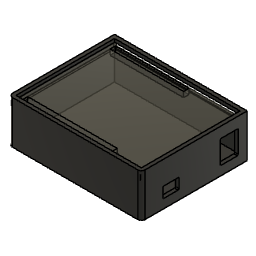
Boite Arduino SATRAGNO (Autodesk Fusion 360 design; units mm, degrees)
Autodesk Fusion 360 part; units mm, degrees
note: some values were not read from the file. Set by a fixed rule: which sketch regions a step uses.
sketch "Esquisse1" plane through (0, 0, 0) normal (0, 1, 0) x (1, 0, 0)
  line L0 (47.3891, -62.8881) -> (-22.6109, -62.8881)
  line L1 (-24.6109, -60.8881) -> (-24.6109, -3.8881)
  line L2 (-24.6109, -3.8881) -> (49.3891, -3.8881)
  line L3 (49.3891, -3.8881) -> (49.3891, -60.8881)
  line L4 (-22.6109, -5.8881) -> (47.3891, -5.8881)
  line L5 (47.3891, -60.8881) -> (-22.6109, -60.8881)
  arc A0 (47.3891, -62.8881) -> (49.3891, -60.8881) centre (47.3891, -60.8881) ccw
  arc A1 (-24.6109, -60.8881) -> (-22.6109, -62.8881) centre (-22.6109, -60.8881) ccw
  line L6 (-22.6109, -5.8881) -> (-22.6109, -60.8881)
  line L7 (47.3891, -5.8881) -> (47.3891, -60.8881)
  point P0 (49.3891, -62.8881)
  point P1 (-24.6109, -62.8881)
  dimension "LongeurCarte" = 74
  dimension "LargeurCrate" = 59
  dimension "d66" = 2
  dimension "d67" = 2
  constraint horizontal L0
  constraint vertical L1
  constraint horizontal L2
  constraint vertical L3
  constraint coincident P0 L0
  constraint coincident P0 L3
  constraint tangent L0 A0
  constraint tangent L3 A0
  constraint coincident P1 L0
  constraint coincident P1 L1
  constraint tangent L0 A1
  constraint tangent L1 A1
  constraint perpendicular L5 L6
  constraint coincident L5.start A0.centre
  constraint perpendicular L5 L7
  measures "LongeurCarte" distance of P0 P1
  measures "LargeurCrate" distance of P1 L1.end
  measures "d66" radius of A0
  measures "d67" radius of A1
extrude "Extrusion5" add sketch "Esquisse1" along normal blind 3 contours L4 L5 L6 L7 makes body 1
extrude "Extrusion6" add sketch "Esquisse1" along normal blind 24 bodies 1
sketch "Esquisse3" plane through (49.3891, 0, 0) normal (1, 0, 0) x (0, 0, -1)
  line L0 (-60.8881, 0) -> (-3.8881, 0)
  line L1 (-3.8881, 0) -> (-3.8881, 24)
  line L2 (-3.8881, 24) -> (-60.8881, 24)
  line L3 (-18.3881, 5) -> (-9.3881, 5)
  line L4 (-18.8881, 5) -> (-18.8881, 0) construction
  line L5 (-18.8881, 5.5) -> (-18.8881, 17.5)
  line L6 (-18.3881, 18) -> (-9.3881, 18)
  line L7 (-8.8881, 17.5) -> (-8.8881, 5.5)
  line L8 (-62.8881, 5) -> (-50.8881, 5) construction
  line L9 (-50.3881, 5) -> (-42.3881, 5)
  line L10 (-3.8881, 0) -> (-60.8881, 0)
  line L11 (-41.8881, 5.5) -> (-41.8881, 10.5)
  line L12 (-42.3881, 11) -> (-50.3881, 11)
  line L13 (-50.8881, 10.5) -> (-50.8881, 5.5)
  arc A0 (-18.3881, 18) -> (-18.8881, 17.5) centre (-18.3881, 17.5) ccw
  arc A1 (-8.8881, 17.5) -> (-9.3881, 18) centre (-9.3881, 17.5) ccw
  arc A2 (-9.3881, 5) -> (-8.8881, 5.5) centre (-9.3881, 5.5) ccw
  arc A3 (-18.8881, 5.5) -> (-18.3881, 5) centre (-18.3881, 5.5) ccw
  arc A4 (-41.8881, 10.5) -> (-42.3881, 11) centre (-42.3881, 10.5) ccw
  arc A5 (-42.3881, 5) -> (-41.8881, 5.5) centre (-42.3881, 5.5) ccw
  arc A6 (-50.8881, 5.5) -> (-50.3881, 5) centre (-50.3881, 5.5) ccw
  arc A7 (-50.3881, 11) -> (-50.8881, 10.5) centre (-50.3881, 10.5) ccw
  line L14 (-60.8881, 24) -> (-60.8881, 0)
  point P0 (-3.8881, 5)
  point P1 (-18.8881, 18)
  point P2 (-8.8881, 18)
  point P3 (-41.8881, 5)
  point P4 (-41.8881, 11)
  point P5 (-50.8881, 11)
  dimension "d18" = 15
  dimension "d19" = 5
  dimension "d20" = 13
  dimension "d21" = 10
  dimension "d22" = 12
  dimension "d23" = 9
  dimension "d24" = 5
  dimension "d25" = 6
  dimension "d26" = 9
  dimension "d27" = 0.5
  dimension "d28" = 0.5
  dimension "d29" = 0.5
  dimension "d30" = 0.5
  dimension "d31" = 0.5
  dimension "d32" = 0.5
  dimension "d33" = 0.5
  dimension "d34" = 0.5
  constraint coincident L1 P0
  constraint perpendicular L1 L3
  constraint coincident L0 L4.end
  constraint perpendicular L0 L4
  constraint perpendicular L3 L5
  constraint perpendicular L5 L6
  constraint perpendicular L3 L7
  constraint perpendicular L9 L11
  constraint perpendicular L11 L12
  constraint coincident P1 L5
  constraint coincident P1 L6
  constraint tangent L5 A0
  constraint tangent L6 A0
  constraint coincident P2 L6
  constraint coincident P2 L7
  constraint tangent L6 A1
  constraint tangent L7 A1
  constraint coincident P0 L3
  constraint tangent L3 A2
  constraint tangent L7 A2
  constraint coincident L4.start L5
  constraint coincident L4.start L3
  constraint tangent L5 A3
  constraint tangent L3 A3
  constraint coincident P4 L12
  constraint coincident P4 L11
  constraint tangent L12 A4
  constraint tangent L11 A4
  constraint coincident P3 L11
  constraint coincident P3 L9
  constraint tangent L11 A5
  constraint tangent L9 A5
  constraint coincident L8.end L13
  constraint coincident L8.end L9
  constraint tangent L13 A6
  constraint tangent L9 A6
  constraint coincident P5 L12
  constraint coincident P5 L13
  constraint tangent L12 A7
  constraint tangent L13 A7
  measures "d18" distance of L4.start P0
  measures "d19" distance of L4.start L4.end
  measures "d20" distance of L4.start P1
  measures "d21" distance of P1 P2
  measures "d22" distance of L8.start L8.end
  measures "d23" distance of L8.end P3
  measures "d24" distance of P3 L10
  measures "d25" distance of P3 P4
  measures "d26" distance of P4 P5
  measures "d27" radius of A0
  measures "d28" radius of A1
  measures "d29" radius of A2
  measures "d30" radius of A3
  measures "d31" radius of A4
  measures "d32" radius of A5
  measures "d33" radius of A6
  measures "d34" radius of A7
extrude "Extrusion7" cut sketch "Esquisse3" against normal blind 2 contours L3 L5 L6 L7 A0 A1 A2 A3 | L9 L11 L12 L13 A4 A5 A6 A7 bodies 1
sketch "Esquisse4" plane through (0, 0, 0) normal (0, 1, 0) x (1, 0, 0)
  line L0 (-73.5353, -62.2391) -> (-145.5353, -62.2391)
  line L1 (-145.5353, -62.2391) -> (-145.5353, -5.2391)
  line L2 (-145.5353, -5.2391) -> (-73.5353, -5.2391)
  line L3 (-73.5353, -5.2391) -> (-73.5353, -62.2391)
  line L4 (-142.5353, -7.2391) -> (-101.5353, -7.2391)
  line L5 (-101.5353, -7.2391) -> (-101.5353, -10.2391)
  line L6 (-101.5353, -10.2391) -> (-142.5353, -10.2391)
  line L7 (-142.5353, -10.2391) -> (-142.5353, -7.2391)
  line L8 (-142.5353, -59.2391) -> (-92.5353, -59.2391)
  line L9 (-92.5353, -59.2391) -> (-92.5353, -56.2391)
  line L10 (-92.5353, -56.2391) -> (-142.5353, -56.2391)
  line L11 (-142.5353, -56.2391) -> (-142.5353, -59.2391)
  dimension "d37" = 72
  dimension "d38" = 57
  dimension "d41" = 41
  dimension "d42" = 3
  dimension "d44" = 50
  dimension "d45" = 3
  constraint horizontal L0
  constraint vertical L1
  constraint horizontal L2
  constraint vertical L3
  constraint horizontal L4
  constraint vertical L5
  constraint horizontal L6
  constraint vertical L7
  constraint horizontal L8
  constraint vertical L9
  constraint horizontal L10
  constraint vertical L11
  measures "d37" distance of L0.start L0.end
  measures "d38" distance of L0.end L1.end
  measures "d41" distance of L5.end L6.end
  measures "d42" distance of L4.start L6.end
  measures "d44" distance of L8.start L8.end
  measures "d45" distance of L8.start L10.end
extrude "Extrusion8" add sketch "Esquisse4" along normal blind 3 separate body makes body 2
sketch "Esquisse5" plane through (0, 0, 3.8881) normal (0, 0, -1) x (-1, 0, 0)
  line L0 (-49.3891, 0) -> (24.6109, 0)
  line L1 (24.6109, 0) -> (24.6109, 24)
  line L2 (24.6109, 24) -> (-49.3891, 24)
  line L3 (-49.3891, 24) -> (-49.3891, 0)
  line L4 (23.6109, 22.1705) -> (23.6109, 21)
  line L5 (23.6109, 21) -> (23.6109, 22.1705)
  line L6 (23.6109, 21) -> (23.6272, 21)
  line L7 (-48.3891, 18.9705) -> (23.6272, 18.9705)
  line L8 (23.6272, 18.9705) -> (23.6272, 22.1705)
  line L9 (23.6272, 22.1705) -> (-48.3891, 22.1705)
  line L10 (-48.3891, 22.1705) -> (-48.3891, 18.9705)
  dimension "d54" = 3.2
  dimension "d86" = 72.0162
  constraint perpendicular L2 L4
  constraint perpendicular L1 L6
  constraint horizontal L7
  constraint vertical L8
  constraint horizontal L9
  constraint vertical L10
  constraint coincident L9 L4.start
  constraint coincident L8 L6.end
  measures "d54" distance of L7.start L9.end
  measures "d86" distance of L7.start L7.end
extrude "Extrusion9" cut sketch "Esquisse5" against normal blind 58 contours L4 L5 L6 L7 L8 L9 L10 bodies 1
copy_body "Corps->Comp1" bodies 2 removing the originals makes body 3 in component "Plexi"
copy_body "Corps->Comp2" bodies 1 removing the originals makes body 4 in component "Boite"
component "Plexi" placed x (1, 0, 0) y (0, 1, 0) z (0, 0, 1) at (121.9244, 19.1705, 0.1489)
component "Boite" placed x (1, 0, 0) y (0, 1, 0) z (0, 0, 1) at (0, 0, 0)
equation "LongeurCarte = LongueurCarte"
equation "LargeurCrate = LargeurCarte"
equation "HauteurBoite = 24 mm"
equation "HauteurFond = 3 mm"
equation "d16 = HauteurBoite"
equation "d54 = HauteurPlexiJeu"
equation "d66 = Coin"
equation "d67 = Coin"
equation "largeursupport = 1 mm"
equation "LongueurCarte = 74.00 mm"
equation "LargeurCarte = 59.00 mm"
equation "Hauteur_Fond = 3.00 mm"
equation "Hauteur_Boite = 24.00 mm"
equation "Coin = 2 mm"
equation "d86 = LongeurPLexiJeu"
equation "LongeurPLexiJeu = 72.016224 mm"
equation "HauteurPlexiJeu = 3.2 mm"
